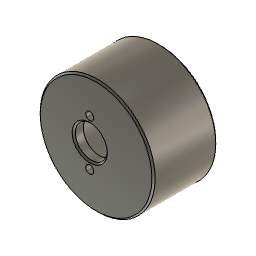
モーターマウント(内部) (Autodesk Fusion 360 design; units mm, degrees)
Autodesk Fusion 360 part; units mm, degrees
sketch "スケッチ1" plane through (0, 0, 0) normal (0, 1, 0) x (1, 0, 0)
  circle A0 centre (0, 0) radius 18
  circle A1 centre (-2, 0) radius 13.85
  dimension "d5" = 27.7
  constraint coincident A0.centre origin
  measures "d5" diameter of A1
extrude "押し出し2" add sketch "スケッチ1" along normal blind 20
sketch "スケッチ2" plane through (0, 0, 0) normal (0, 1, 0) x (1, 0, 0)
  circle A0 centre (-2, 0) radius 13.85
  circle A1 centre (-2, 0) radius 5
  dimension "d8" = 27.7
  dimension "d11" = 10
  constraint concentric A0 A1
  measures "d8" diameter of A0
  measures "d11" diameter of A1
extrude "押し出し4" add sketch "スケッチ2" along normal blind 3
sketch "スケッチ3" plane through (0, 0, 0) normal (0, -1, 0) x (1, 0, 0)
  circle A0 centre (-2, 0) radius 5
  circle A1 centre (0, 0) radius 18
  circle A2 centre (-2, -7.25) radius 1.25
  line L0 (-2, 0) -> (-2, 7.25)
  circle A3 centre (-2, 7.25) radius 1.25
  point P0 (-2, 0)
  dimension "d14" = 7.25
  dimension "d15" = 2.5
  dimension "d16" = 7.25
  dimension "d17" = 2.5
  constraint coincident P0 A0.centre
  constraint vertical L0
  constraint coincident L0.end A3.centre
  measures "d14" distance of P0 A2.centre
  measures "d15" diameter of A2
  measures "d16" distance of P0 L0.end
  measures "d17" diameter of A3
extrude "押し出し5" cut sketch "スケッチ3" against normal blind 3 contours A2 | A3
chamfer "面取り1" distance 0.5 angle 45 2 edges at (-16.7819, 0, 6.5091) (-6.6616, 0, -1.8081)
chamfer "面取り2" distance 0.5 angle 45 2 edges at (-16.7819, 20, 6.5091) (-14.9127, 20, -5.0084)
sketch "スケッチ4" plane through (0, 0, 0) normal (0, 1, 0) x (1, 0, 0)
